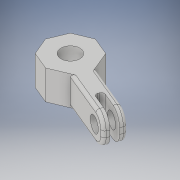
# Autodesk Inventor part: Hex_Center
Saved by Autodesk Inventor 2019 (Build 230136000, 136)
## iProperties
Created: 2019-11-16
Part Number: Hex_Center
Material: Generic
Document SubType Name: Modeling
Designer: Jorian Brusind
Density: 1 g/cm^3
Appearance: Default
Author: Jorian Brusind
Autodesk Inventor part; units mm, degrees
ref_plane "YZ Plane" through (0, 0, 0) normal (1, 0, 0) x (0, 1, 0)
ref_plane "XZ Plane" through (0, 0, 0) normal (0, 1, 0) x (-1, 0, 0)
ref_plane "XY Plane" through (0, 0, 0) normal (0, 0, 1) x (1, 0, 0)
sketch "Sketch6" plane through (0, 0, 0) normal (0, 1, 0) x (-1, 0, 0)
  line L0 (4.2426, 0) -> (3, -3)
  line L1 (3, -3) -> (0, -4.2426)
  line L2 (0, -4.2426) -> (-3, -3)
  line L3 (-3, -3) -> (-4.2426, 0)
  line L4 (-4.2426, 0) -> (-3, 3)
  line L5 (-3, 3) -> (0, 4.2426)
  line L6 (0, 4.2426) -> (3, 3)
  line L7 (3, 3) -> (4.2426, 0)
  point P0 (0, 0)
  point P1 (0, 0)
  dimension "d38" = 3
  dimension "d39" = 3
  constraints: 16 end point, 1 coincident, 17 other
  measures "d38" vertical distance of L0.start L0.end
  measures "d39" vertical distance of L6.end L0.start
extrude "Extrusion7" add sketch "Sketch6" along normal blind 5
sketch "Sketch7" plane through (4.2426, 0, 0) normal (0.9238795, 0, 0.3826834) x (0.3826834, 0, -0.9238795)
  line L0 (-3.2472, 5) -> (0, 5) projected
  line L1 (0, 0) -> (0, 5) projected
  line L2 (-3.2472, 5) -> (0, 5)
  line L3 (0, 5) -> (0, 0)
  line L4 (0, 0) -> (-3.2472, 0)
  line L5 (-3.2472, 0) -> (-3.2472, 5)
  point P0 (-1.6236, 0)
  constraints: 8 end point, 2 parallel, 1 horizontal, 1 perpendicular
extrude "Extrusion8" add sketch "Sketch7" along normal blind 10
sketch "Sketch8" plane through (13.4814, 0, 3.8268) normal (0.9238795, 0, 0.3826834) x (0.3826834, 0, -0.9238795)
  line L0 (-1.6236, 0) -> (-1.6236, 2.5)
  line L1 (-0.9986, 0) -> (-2.2486, 0)
  line L2 (-2.2486, 0) -> (-2.2486, 5)
  line L3 (-2.2486, 5) -> (-0.9986, 5)
  line L4 (-0.9986, 5) -> (-0.9986, 0)
  line L5 (-0.9986, 0) -> (-2.2486, 5) construction
  line L6 (-2.2486, 0) -> (-0.9986, 5) construction
  dimension "d44" = 2.5
  dimension "d45" = 1.25
  dimension "d46" = 5
  constraints: 14 end point, 2 midpoint, 2 parallel, 1 horizontal, 1 perpendicular, 1 vertical
  measures "d44" distance of L0.start L0.end
  measures "d45" distance of L2.end L3.end
  measures "d46" distance of L1.end L2.end
extrude "Extrusion9" cut sketch "Sketch8" against normal blind 5
sketch "Sketch9" plane through (4.2426, 0, 0) normal (0.3826834, 0, -0.9238795) x (-0.9238795, 0, -0.3826834)
  line L0 (0, 5) -> (-10, 5) projected
  line L1 (-10, 5) -> (-7.5, 5)
  line L2 (-7.5, 5) -> (-7.5, 2.5)
  circle A0 centre (-7.5, 2.5) radius 1.25
  point P0 (3.9197, 0)
  dimension "d49" = 2.5
  dimension "d50" = 2.5
  dimension "d51" = 2.5
  constraints: 4 end point, 1 centre point, 1 coincident, 1 perpendicular, 1 point on line
  measures "d49" distance of L0.end L1.end
  measures "d50" distance of L1.end L2.end
  measures "d51" diameter of A0
extrude "Extrusion10" cut sketch "Sketch9" against normal blind 4
fillet "Fillet2" radius 2 4 edges at (13.2904, 5, 4.2881) (12.4299, 5, 6.3655) (12.4299, 0, 6.3655) (13.2904, 0, 4.2881)
fillet "Fillet3" radius 0.5 2 edges at (7.9997, 2.5, 3.9901) (8.478, 2.5, 2.8352)
fillet "Fillet4" radius 0.5 10 edges at (12.9402, 4.4142, 3.6027) (13.4814, 2.5, 3.8268) (12.9402, 0.5858, 3.6027) (7.9382, 0, 1.5307) (7.9382, 5, 1.5307) (11.6976, 4.4142, 6.6027) (12.2388, 2.5, 6.8268) (11.6976, 0.5858, 6.6027) (6.6955, 0, 4.5307) (6.6955, 5, 4.5307)
sketch "Sketch10" plane through (0, 5, 0) normal (0, 1, 0) x (1, 0, 0)
  circle A0 centre (0, 0) radius 1.6
  dimension "d57" = 3.2
  constraints: 1 centre point, 1 coincident
  measures "d57" diameter of A0
extrude "Extrusion11" cut sketch "Sketch10" against normal blind 5
body "Solid2"
